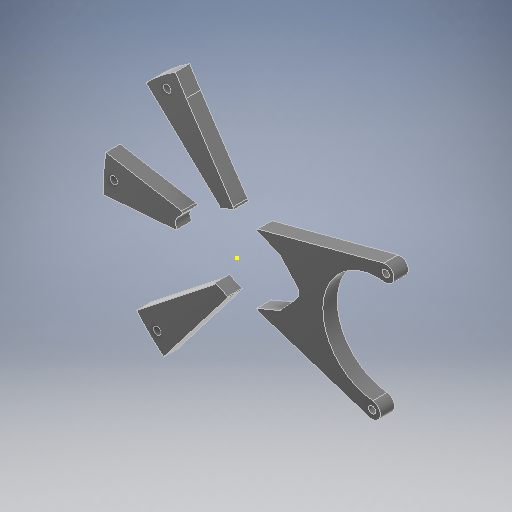
# Autodesk Inventor part: MotorConnectionRoundyBit
Saved by Autodesk Inventor 2026.1 (Build 301233000, 233)
## iProperties
Created: 2025-10-13
Part Number: MotorConnectionRoundyBit
Material: Plastic, Opaque Black
Document SubType Name: Modeling
Designer: Teddy
Density: 0.952 g/cm^3
Appearance: Smooth - Black
Author: Teddy
Autodesk Inventor part; units mm, degrees
ref_plane "YZ Plane" through (0, 0, 0) normal (1, 0, 0) x (0, 1, 0)
ref_plane "XZ Plane" through (0, 0, 0) normal (0, 1, 0) x (-1, 0, 0)
ref_plane "Work Plane1" through (0, 0, 0) normal (0, 0, 1) x (1, 0, 0)
sketch "Sketch1" plane through (0, 0, 0) normal (0, 0, 1) x (1, 0, 0)
  circle A0 centre (33.02, 0) radius 2.286
  circle A1 centre (-33.02, 0) radius 2.286
  circle A2 centre (0, 20.32) radius 2.286
  circle A3 centre (0, -20.32) radius 2.286
  arc A4 (-27.8119, -10.2) -> (-26.3675, -11.6445) centre (-26.3675, -10.2) ccw
  line L0 (-26.3675, -11.6445) -> (-25.45, -11.6445)
  arc A5 (-23.5945, -13.5) -> (-25.45, -11.6445) centre (-25.45, -13.5) ccw
  line L1 (-23.5945, -13.5) -> (-23.5945, -14.2175)
  arc A6 (-23.5945, -14.2175) -> (-22.452, -15.63) centre (-22.15, -14.2175) ccw
  line L2 (-22.452, -15.63) -> (-22.452, -15.827)
  line L3 (-22.452, -15.827) -> (-21.448, -15.827)
  line L4 (-21.448, -15.827) -> (-21.448, -15.6619)
  line L5 (-21.448, -15.6619) -> (22.15, -15.6619)
  arc A7 (22.15, -15.6619) -> (23.5945, -14.2175) centre (22.15, -14.2175) ccw
  line L6 (23.5945, -14.2175) -> (23.5945, -13.5)
  arc A8 (25.45, -11.6445) -> (23.5945, -13.5) centre (25.45, -13.5) ccw
  line L7 (25.45, -11.6445) -> (26.3675, -11.6445)
  arc A9 (26.3675, -11.6445) -> (27.8119, -10.2) centre (26.3675, -10.2) ccw
  line L8 (27.8119, -10.2) -> (27.8119, 10.2)
  arc A10 (27.8119, 10.2) -> (26.3675, 11.6445) centre (26.3675, 10.2) ccw
  line L9 (26.3675, 11.6445) -> (25.45, 11.6445)
  arc A11 (23.5945, 13.5) -> (25.45, 11.6445) centre (25.45, 13.5) ccw
  line L10 (23.5945, 13.5) -> (23.5945, 14.2175)
  arc A12 (23.5945, 14.2175) -> (22.15, 15.6619) centre (22.15, 14.2175) ccw
  line L11 (22.15, 15.6619) -> (-21.448, 15.6619)
  line L12 (-21.448, 15.6619) -> (-21.448, 15.827)
  line L13 (-21.448, 15.827) -> (-22.452, 15.827)
  line L14 (-22.452, 15.827) -> (-22.452, 15.63)
  arc A13 (-22.452, 15.63) -> (-23.5945, 14.2175) centre (-22.15, 14.2175) ccw
  line L15 (-23.5945, 14.2175) -> (-23.5945, 13.5)
  arc A14 (-25.45, 11.6445) -> (-23.5945, 13.5) centre (-25.45, 13.5) ccw
  line L16 (-25.45, 11.6445) -> (-26.3675, 11.6445)
  arc A15 (-26.3675, 11.6445) -> (-27.8119, 10.2) centre (-26.3675, 10.2) ccw
  line L17 (-27.8119, 10.2) -> (-27.8119, -10.2)
  arc A16 (-27.7187, -15.3162) -> (-26.4301, -16.225) centre (-25.05, -12.9) ccw
  line L18 (-27.7187, -15.3162) -> (-37.7272, -4.262)
  arc A17 (-37.7272, 4.262) -> (-37.7272, -4.262) centre (-33.02, 0) ccw
  line L19 (-37.7272, 4.262) -> (-27.7187, 15.3162)
  arc A18 (-26.4301, 16.225) -> (-27.7187, 15.3162) centre (-25.05, 12.9) ccw
  line L20 (-26.4301, 16.225) -> (-2.4343, 26.1849)
  arc A19 (2.4343, 26.1849) -> (-2.4343, 26.1849) centre (0, 20.32) ccw
  line L21 (2.4343, 26.1849) -> (26.4301, 16.225)
  arc A20 (27.7187, 15.3162) -> (26.4301, 16.225) centre (25.05, 12.9) ccw
  line L22 (27.7187, 15.3162) -> (37.7272, 4.262)
  arc A21 (37.7272, -4.262) -> (37.7272, 4.262) centre (33.02, 0) ccw
  line L23 (37.7272, -4.262) -> (27.7187, -15.3162)
  arc A22 (26.4301, -16.225) -> (27.7187, -15.3162) centre (25.05, -12.9) ccw
  line L24 (26.4301, -16.225) -> (2.4343, -26.1849)
  arc A23 (-2.4343, -26.1849) -> (2.4343, -26.1849) centre (0, -20.32) ccw
  line L25 (-2.4343, -26.1849) -> (-26.4301, -16.225)
  circle A24 centre (-76.1268, 3.6068) radius 2.286
  arc A25 (-81.1848, 16.0688) -> (-82.2658, -7.3525) centre (12.7, 0) ccw
  line L26 (-68.6668, 13.9263) -> (-81.1848, 16.0688)
  arc A26 (-68.6668, 13.9263) -> (-69.6037, -6.3721) centre (12.7, 0) ccw
  line L27 (-82.2658, -7.3525) -> (-69.6037, -6.3721)
  circle A27 centre (-43.2949, 69.0491) radius 2.286
  arc A28 (-38.1798, 80.5221) -> (-56.3085, 65.6536) centre (12.7, 0) ccw
  line L28 (-31.3958, 69.7858) -> (-38.1798, 80.5221)
  arc A29 (-31.3958, 69.7858) -> (-47.1073, 56.8998) centre (12.7, 0) ccw
  line L29 (-56.3085, 65.6536) -> (-47.1073, 56.8998)
  circle A30 centre (-49.4171, -63.5977) radius 2.286
  circle A31 centre (-49.4171, -63.5977) radius 2.286
  arc A32 (-62.0626, -59.0179) -> (-45.3806, -75.4931) centre (12.7, 0) ccw
  line L30 (-52.0943, -51.1489) -> (-62.0626, -59.0179)
  arc A33 (-52.0943, -51.1489) -> (-37.6365, -65.4274) centre (12.7, 0) ccw
  line L31 (-45.3806, -75.4931) -> (-37.6365, -65.4274)
  line L32 (-31.3958, 69.7858) -> (-2.4343, 26.1849)
  line L33 (-47.1073, 56.8998) -> (-11.0598, 22.6047)
  line L34 (-68.6668, 13.9263) -> (-34.3024, 8.0446)
  line L35 (-69.6037, -6.3721) -> (-38.0108, -3.9261)
  line L36 (-37.6365, -65.4274) -> (-6.2324, -24.6084)
  line L37 (-52.0943, -51.1489) -> (-14.2551, -21.2784)
  circle A34 centre (83.416, -39.4819) radius 2.1844
  circle A35 centre (91.9268, 37.6997) radius 2.1844
  circle A36 centre (91.9268, 37.6997) radius 5.08
  circle A37 centre (83.416, -39.4819) radius 5.08
  arc A38 (91.2509, 32.6649) -> (83.8534, -34.4207) centre (86.7596, -0.7905) ccw
  line L38 (90.6234, 42.6097) -> (12.7, 21.9239)
  line L39 (81.8511, -44.3148) -> (12.7, -21.9239)
  point P0 (0, 0)
extrude "Extrusion1" add sketch "Sketch1" against normal blind 8.89 contours L25 L36 A33 L37 | L35 A26 L34 L19 A17 | A33 L31 A32 L30 | L27 A25 L26 A26 | L24 A22 L23 A21 L22 A20 L21 L38 A36 A38 A37 L39 | A37 | L33 A29 L32 L20 | L29 A28 L28 A29 | A36
sketch "Sketch2" plane through (0, 0, 0) normal (0, 0, 1) x (1, 0, 0)
  point P0 (0, 0)
thicken "Thicken1" operation add thickness 1.27 both sides no extend neighbours no toward (0.7912881, -0.6114435, 0) faces at (-38.0447, 3.8827, -5.9267) (-36.5856, 5.5229, -2.9633)
thicken "Thicken2" operation add thickness 1.27 both sides no extend neighbours no toward (0.3833577, -0.9235999, 0) faces at (-8.1846, 23.7981, -2.9633)
thicken "Thicken3" operation add thickness 1.27 both sides no extend neighbours no toward (-0.3833577, -0.9235999, 0) faces at (17.2767, 20.0242, -2.9633) (27.597, 15.4442, -5.9267) (31.0549, 11.6315, -2.9633) (38.8468, -2.524, -5.9267) (34.3911, -7.9467, -5.9267) (27.597, -15.4442, -2.9633) (21.8534, -18.1246, -2.9633)
thicken "Thicken4" operation add thickness 1.27 both sides no extend neighbours no toward (0.3833577, 0.9235999, 0) faces at (-8.9066, -23.4984, -2.9633)
body "Solid1"
